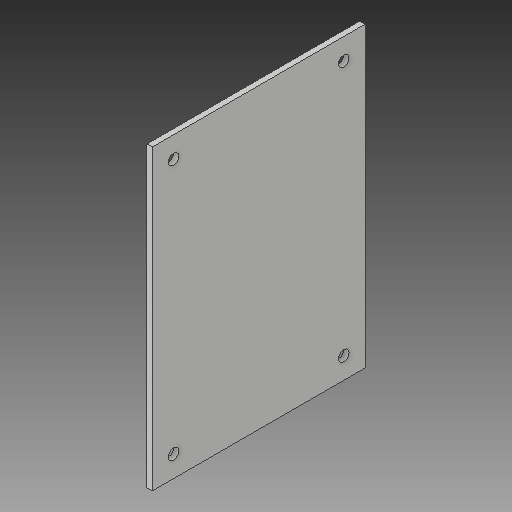
# Autodesk Inventor part: 1512898-16-P-0701
Saved by Autodesk Inventor 2017 (Build 210142000, 142)
## iProperties
Created: 2016-10-09
Part Number: 1512898-16-P-0701
Material: Generic
Document SubType Name: Modeling
Designer: gus
Density: 1 g/cm^3
Appearance: Default
Mass: 71.2912 g
Surface Area: 470.967 cm^2
Volume: 71.2912 cm^3
Author: gus
Autodesk Inventor part; units mm, degrees
ref_plane "YZ Plane" through (0, 0, 0) normal (1, 0, 0) x (0, 1, 0)
ref_plane "XZ Plane" through (0, 0, 0) normal (0, 1, 0) x (-1, 0, 0)
ref_plane "XY Plane" through (0, 0, 0) normal (0, 0, 1) x (1, 0, 0)
sketch "Sketch1" plane through (0, 0, 0) normal (1, 0, 0) x (0, 1, 0)
  line L0 (0, 0) -> (177.8, 0)
  line L1 (177.8, 0) -> (177.8, -127)
  line L2 (177.8, -127) -> (0, -127)
  line L3 (0, -127) -> (0, 0)
  circle A0 centre (12.7, -12.7) radius 3.175
  circle A1 centre (165.1, -12.7) radius 3.175
  circle A2 centre (12.7, -114.3) radius 3.175
  circle A3 centre (165.1, -114.3) radius 3.175
  dimension "d0" = 12.7
  dimension "d1" = 12.7
  dimension "d2" = 12.7
  dimension "d3" = 12.7
  dimension "d4" = 12.7
  dimension "d5" = 12.7
  dimension "d6" = 12.7
  dimension "d7" = 12.7
  dimension "d8" = 152.4
  dimension "d9" = 101.6
  dimension "d10" = 6.35
  constraints: 8 end point, 4 centre point, 3 equal radius, 2 parallel, 1 horizontal, 1 perpendicular
  measures "d0" distance from line of L2 A2.centre
  measures "d1" distance from line of L3 A2.centre
  measures "d2" distance from line of L3 A0.centre
  measures "d3" distance from line of L0 A0.centre
  measures "d4" distance from line of L0 A1.centre
  measures "d5" distance from line of L1 A1.centre
  measures "d6" distance from line of L2 A3.centre
  measures "d7" distance from line of L1 A3.centre
  measures "d8" distance of A3.centre A2.centre
  measures "d9" distance of A0.centre A2.centre
  measures "d10" diameter of A2
extrude "Extrusion1" add sketch "Sketch1" along normal blind 3.175
body "Solid1"
